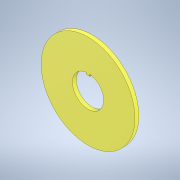
# Autodesk Inventor part: 6x1_4-testSampleGear
Saved by Autodesk Inventor 2021.1 (Build 251245010, 245A)
## iProperties
Created: 2020-11-07
Part Number: 6x1_4-testSampleGear
Material: PC/ABS Plastic
Document SubType Name: Modeling
Designer: robst
Density: 0.357273 g/cm^3
Appearance: Smooth - Yellow
Author: robst
Autodesk Inventor part; units mm, degrees
ref_plane "YZ Plane" through (0, 0, 0) normal (1, 0, 0) x (0, 1, 0)
ref_plane "XZ Plane" through (0, 0, 0) normal (0, 1, 0) x (-1, 0, 0)
ref_plane "XY Plane" through (0, 0, 0) normal (0, 0, 1) x (1, 0, 0)
sketch "Sketch1" plane through (0, 0, 0) normal (0, 0, 1) x (1, 0, 0)
  circle A0 centre (0, 0) radius 76.2
  dimension "d0" = 152.4
  constraints: 1 centre point, 1 coincident
  measures "d0" diameter of A0
extrude "Extrusion1" add sketch "Sketch1" along normal mid plane 6.35
sketch "Sketch3" plane through (0, 0, 3.175) normal (0, 0, 1) x (1, 0, 0)
  circle A0 centre (0, 0) radius 25.4
  dimension "d8" = 50.8
  constraints: 1 centre point, 1 coincident
  measures "d8" diameter of A0
extrude "Extrusion3" cut sketch "Sketch3" against normal through all
sketch "Sketch5" plane through (0, 0, 3.175) normal (0, 0, 1) x (1, 0, 0)
  arc A0 (3.175, 25.2008) -> (-3.175, 25.2008) centre (0, 0) ccw
  circle A1 centre (0, 0) radius 25.4 projected
  line L0 (-3.175, 25.2008) -> (-3.175, 22.225)
  line L1 (3.175, 25.2008) -> (3.175, 22.225)
  line L2 (-3.175, 22.225) -> (3.175, 22.225)
  dimension "d11" = 3.175
  dimension "d13" = 6.35
  constraints: 6 end point, 4 point on circle, 2 vertical, 1 centre point, 1 coincident, 1 horizontal, 1 parallel
  measures "d11" distance edge to line of A0 L2
  measures "d13" distance of L1.end L0.end
extrude "Extrusion4" add sketch "Sketch5" against normal blind 6.35 contours L1 L2 L0 A0
sketch "Sketch7" plane through (0, 0, -3.175) normal (0, 0, -1) x (-1, 0, 0)
  arc A0 (3.175, -25.2008) -> (20.237, -15.35) centre (0, 0) ccw projected
  circle A1 centre (0, 0) radius 38.1
  circle A2 centre (0, 0) radius 4.7625
  dimension "d19" = 76.2
  dimension "d20" = 9.525
  constraints: 2 centre point, 2 coincident
  measures "d19" diameter of A1
  measures "d20" diameter of A2
body "Solid1"
